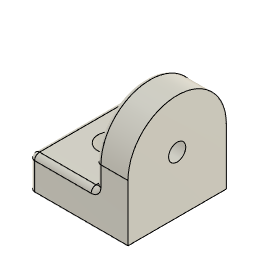
Webcam holder 2020 extrusion mount x2 (Autodesk Fusion 360 design; units mm, degrees)
Autodesk Fusion 360 part; units mm, degrees
sketch "Sketch1" plane through (0, 0, 0) normal (0, 0, 1) x (1, 0, 0)
  line L0 (0, 0) -> (20, 0)
  line L1 (20, 0) -> (20, 20)
  line L2 (20, 20) -> (0, 20)
  line L3 (0, 20) -> (0, 0)
  dimension "d34" = 20
  constraint horizontal L0
  constraint vertical L1
  constraint horizontal L2
  constraint vertical L3
  constraint coincident L0.start L3.end
  measures "d34" distance of L1.end L2.end
extrude "Extrude1" add sketch "Sketch1" along normal blind 6.5
sketch "Sketch2" plane through (0, 0, 6.5) normal (0, 0, 1) x (-1, 0, 0)
  line L0 (0, -20) -> (0, 0)
  line L1 (0, 0) -> (-20, 0)
  line L2 (-20, 0) -> (-20, -20)
  line L3 (-20, -20) -> (0, -20)
  line L4 (-20, -20) -> (-20, 0)
  line L5 (-13.5, 0) -> (-13.5, -20)
  line L6 (-13.5, -20) -> (0, 0) construction
  dimension "d33" = 6.5
  constraint coincident L2.end L3.start
  constraint coincident L1.end L2.start
  constraint coincident L1 L5.start
  constraint coincident L3 L5.end
  constraint perpendicular L3 L5
  constraint coincident L0.end L1.start
  measures "d33" distance of L4 L5
extrude "Extrude2" add sketch "Sketch2" along normal blind 15 contours L1 L2 L3 L4 L5
sketch "Sketch5" plane through (20, 0, 0) normal (1, 0, 0) x (0, 1, 0)
  line L0 (0, 21.5) -> (0, 0)
  line L1 (0, 0) -> (20, 0)
  line L2 (20, 0) -> (20, 21.5)
  line L3 (20, 21.5) -> (0, 21.5)
  line L4 (0, 21.5) -> (20, 1.5) construction
  line L5 (0, 21.5) -> (20, 21.5) construction
  line L6 (20, 21.5) -> (10, 11.5) construction
  dimension "d37" = 45
  constraint horizontal L5
  constraint coincident L0.start L3.end
  constraint coincident L2 L4.end
  constraint coincident L2.end L3.start
  constraint midpoint L4 L6.end
  measures "d37" angle of L4 L5
fillet "Fillet2" radius 10 2 edges at (16.75, 20, 21.5) (16.75, 0, 21.5)
hole "Hole3" at (13.5, 10, 11.5) direction (1, 0, 0) diameter 3.5 end through all counterbore diameter 5.7 counterbore depth 3.5
hole "Hole4" at (6.75, 10, 6.5) direction (0, 0, -1) diameter 3.5 end through all counterbore diameter 5.7 counterbore depth 3.5
fillet "Fillet1" radius 1 9 edges at (0, 20, 3.25) (0, 0, 3.25) (6.75, 0, 6.5) (6.75, 20, 6.5) (0, 10, 6.5) (13.5, 20, 9) (13.5, 10, 21.5) (13.5, 0, 9) (13.5, 10, 6.5)
